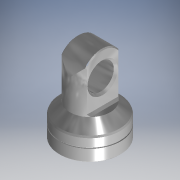
# Autodesk Inventor part: Top
Saved by Autodesk Inventor 2016 (Build 200138000, 138)
## iProperties
Created: 2013-09-01
Part Number: Top
Material: Steel
Document SubType Name: Modeling
Designer: Arto
Density: 7.85 g/cm^3
Appearance: Anodisé - Gris clair
Author: Arto
Autodesk Inventor part; units mm, degrees
ref_plane "YZ Plane" through (0, 0, 0) normal (1, 0, 0) x (0, 1, 0)
ref_plane "XZ Plane" through (0, 0, 0) normal (0, 1, 0) x (-1, 0, 0)
ref_plane "XY Plane" through (0, 0, 0) normal (0, 0, 1) x (1, 0, 0)
sketch "Sketch1" plane through (0, 0, 0) normal (0, 0, 1) x (1, 0, 0)
  circle A0 centre (0, 0) radius 10 construction
  circle A1 centre (0, 0) radius 30
  dimension "d0" = 60
  constraints: 1 centre point, 1 coincident
  measures "d0" diameter of A1
extrude "Extrusion1" add sketch "Sketch1" along normal blind 20
chamfer "Chamfer1" distance 10 angle 45 1 edges at (-30, 0, 20)
sketch "Sketch2" plane through (0, 0, 20) normal (0, 0, 1) x (1, 0, 0)
  circle A0 centre (0, 0) radius 20 projected
  line L0 (12.5, -15.6125) -> (12.5, 15.6125)
  line L1 (-12.5, -15.6125) -> (-12.5, 15.6125)
  dimension "d6" = 25
  constraints: 4 end point, 4 point on circle, 2 parallel, 1 vertical
  measures "d6" distance between parallel lines of L1 L0
extrude "Extrusion2" add sketch "Sketch2" along normal blind 50 contours L0 A0 L1
sketch "Sketch3" plane through (12.5, -15.6125, 20) normal (1, 0, 0) x (0, 0, -1)
  line L0 (-50, 35.6125) -> (-50, 31.225) construction
  line L1 (-50, 0) -> (-50, -4.3875) construction
  arc A0 (-29.8077, 35.9971) -> (-29.8077, -4.3875) centre (-29.8077, 15.8048) ccw
  line L2 (-29.8077, -4.3875) -> (-29.8077, 35.9971) construction
  line L3 (-29.8077, -4.3875) -> (10.5769, -4.3875) construction
  line L4 (-29.8077, -4.3875) -> (-57.4688, -4.3875)
  line L5 (-57.4688, -4.3875) -> (-57.4688, 35.9971)
  line L6 (-57.4688, 35.9971) -> (-29.8077, 35.9971)
  line L7 (-50, 0) -> (-50, 31.225) construction
  point P0 (20, 15.6125)
  dimension "d9" = 90
  constraints: 10 end point, 2 perpendicular, 2 point on circle, 1 centre point, 1 collinear, 1 horizontal, 1 midpoint, 1 parallel, 1 point on line, 1 tangent
  measures "d9" angle of L3 L2
extrude "Extrusion3" cut sketch "Sketch3" against normal through all
hole "Hole1" at (12.5, 0, 45.897) direction (-1, 0, 0) diameter 26 end through all
chamfer "Chamfer2" distance 1 angle 45 2 edges at (-30, 0, 0) (-30, 0, 10)
chamfer "Chamfer3" distance 2 angle 45 2 edges at (-12.5, 0, 20) (12.5, 0, 20)
chamfer "Chamfer4" distance 1 angle 45 2 edges at (12.5, -0.111, 69.9977) (-12.5, -0.111, 69.9977)
chamfer "Chamfer5" distance 2 angle 45 2 edges at (12.5, 0, 58.897) (-12.5, 0, 58.897)
sketch "Sketch4" plane through (0, 0, 0) normal (0, 0, -1) x (-1, 0, 0)
  circle A0 centre (0, 0) radius 30
  circle A1 centre (0, 0) radius 27
  dimension "d38" = 60
  dimension "d39" = 54
  constraints: 2 centre point, 2 coincident
  measures "d38" diameter of A0
  measures "d39" diameter of A1
extrude "Extrusion4" add sketch "Sketch4" along normal blind 12
chamfer "Chamfer6" distance 5 angle 45 1 edges at (27, 0, 0)
chamfer "Chamfer7" distance 1 angle 45 2 edges at (30, 0, -12) (27, 0, -12)
body "Solid1"
